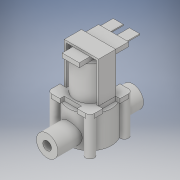
# Autodesk Inventor part: Valve
Saved by Autodesk Inventor 2018 (Build 220112000, 112)
## iProperties
Created: 2019-07-25
Part Number: Valve
Material: Generic
Document SubType Name: Modeling
Designer: micha
Density: 1 g/cm^3
Appearance: Default
Author: micha
Autodesk Inventor part; units mm, degrees
ref_plane "YZ Plane" through (0, 0, 0) normal (1, 0, 0) x (0, 1, 0)
ref_plane "XZ Plane" through (0, 0, 0) normal (0, 1, 0) x (-1, 0, 0)
ref_plane "XY Plane" through (0, 0, 0) normal (0, 0, 1) x (1, 0, 0)
sketch "Sketch1" plane through (0, 0, 0) normal (0, 0, 1) x (1, 0, 0)
  circle A0 centre (0, 0) radius 7.9375
  circle A1 centre (0, 0) radius 3.175
  dimension "d0" = 15.875
  dimension "d1" = 6.35
  constraints: 2 centre point, 2 coincident
  measures "d0" diameter of A0
  measures "d1" diameter of A1
extrude "Extrusion1" add sketch "Sketch1" along normal blind 63.5
sketch "Sketch2" plane through (0, 0, 63.5) normal (0, 0, 1) x (1, 0, 0)
  circle A0 centre (0, 0) radius 7.9375 projected
  point P0 (0, -7.9375)
  constraints: 1 vertical alignment, 1 other
ref_plane "Work Plane1" through (0, -7.9375, 63.5) normal (0, -1, 0) x (1, 0, 0)
sketch "Sketch3" plane through (0, -7.9375, 63.5) normal (0, -1, 0) x (1, 0, 0)
  line L0 (7.9375, 0) -> (-7.9375, 0) projected
  line L1 (0, 0) -> (0, -63.5) construction
  line L2 (-7.9375, -63.5) -> (7.9375, -63.5) projected
  circle A0 centre (0, -31.75) radius 15.875
  dimension "d4" = 31.75
  dimension "d5" = 31.75
  constraints: 2 end point, 2 midpoint, 1 centre point, 1 coincident, 1 vertical
  measures "d4" distance from line of L2 point (0, -31.75)
  measures "d5" diameter of A0
extrude "Extrusion2" add sketch "Sketch3" against normal blind 23.8125
sketch "Sketch4" plane through (0, 15.875, 31.75) normal (0, 1, 0) x (1, 0, 0)
  line L0 (-12.7, -12.7) -> (12.7, -12.7)
  line L1 (12.7, -12.7) -> (12.7, 12.7)
  line L2 (12.7, 12.7) -> (-12.7, 12.7)
  line L3 (-12.7, 12.7) -> (-12.7, -12.7)
  circle A0 centre (0, 0) radius 15.875 projected
  line L4 (-12.7, 6.35) -> (-12.7, -6.35)
  line L5 (-12.7, -6.35) -> (-15.875, -6.35)
  line L6 (-15.875, -6.35) -> (-15.875, -12.7)
  line L7 (-12.7, -15.875) -> (-6.35, -15.875)
  line L8 (-6.35, -15.875) -> (-6.35, -12.7)
  line L9 (-12.7, 6.35) -> (-15.875, 6.35)
  line L10 (-15.875, 6.35) -> (-15.875, 12.7)
  line L11 (-12.7, 15.875) -> (-6.35, 15.875)
  line L12 (-6.35, 15.875) -> (-6.35, 12.7)
  line L13 (6.35, 12.7) -> (6.35, 15.875)
  line L14 (6.35, 15.875) -> (12.7, 15.875)
  line L15 (15.875, 12.7) -> (15.875, 6.35)
  line L16 (15.875, 6.35) -> (12.7, 6.35)
  line L17 (6.35, -12.7) -> (6.35, -15.875)
  line L18 (6.35, -15.875) -> (12.7, -15.875)
  line L19 (15.875, -12.7) -> (15.875, -6.35)
  line L20 (15.875, -6.35) -> (12.7, -6.35)
  arc A1 (-15.875, -12.7) -> (-12.7, -15.875) centre (-12.7, -12.7) ccw
  arc A2 (-12.7, 15.875) -> (-15.875, 12.7) centre (-12.7, 12.7) ccw
  arc A3 (15.875, 12.7) -> (12.7, 15.875) centre (12.7, 12.7) ccw
  arc A4 (12.7, -15.875) -> (15.875, -12.7) centre (12.7, -12.7) ccw
  point P0 (0, 31.75)
  point P1 (-15.875, -15.875)
  point P2 (-15.875, 15.875)
  point P3 (15.875, 15.875)
  point P4 (15.875, -15.875)
  dimension "d8" = 25.4
  dimension "d9" = 25.4
  dimension "d10" = 12.7
  dimension "d11" = 12.7
  dimension "d12" = 6.35
  dimension "d13" = 12.7
  dimension "d14" = 3.175
  dimension "d15" = 9.525
  dimension "d16" = 9.525
  dimension "d17" = 9.525
  dimension "d18" = 19.05
  dimension "d19" = 3.175
  dimension "d20" = 12.7
  dimension "d21" = 9.525
  dimension "d22" = 3.175
  dimension "d23" = 9.525
  dimension "d24" = 12.7
  dimension "d25" = 9.525
  dimension "d26" = 3.175
  constraints: 42 end point, 18 point on line, 14 perpendicular, 9 tangent, 8 point on circle, 4 centre point, 3 equal radius, 3 horizontal, 2 parallel
  measures "d8" distance of L2.end L1.end
  measures "d9" distance of L1.end L0.end
  measures "d10" distance from line of L2 A0.centre
  measures "d11" distance from line of L1 A0.centre
  measures "d12" vertical distance of A0.centre L4.start
  measures "d13" distance of L4.start L4.end
  measures "d14" distance of L4.end L5.end
  measures "d15" distance of L5.end point (-15.875, -15.875)
  measures "d16" distance of point (-15.875, -15.875) L7.end
  measures "d17" distance of L9.end point (-15.875, 15.875)
  measures "d18" distance between parallel lines of L12 L1
  measures "d19" distance of L13.start L13.end
  measures "d20" distance between parallel lines of L13 L12
  measures "d21" distance of L13.end point (15.875, 15.875)
  measures "d22" distance of L17.start L17.end
  measures "d23" distance between parallel lines of L15 L17
  measures "d24" distance between parallel lines of L16 L20
  measures "d25" distance between parallel lines of L16 L14
  measures "d26" radius of A1
extrude "Extrusion3" add sketch "Sketch4" along normal blind 3.175 contours L0 A0 L3 L2 L1 | L8 A0 L0 | L0 A0 L17 | A0 L8 L7 A1 L6 L5 L3 L0 | L0 L3 A0 | A0 L1 L0 | L0 L1 A0 L20 L19 A4 L18 L17 | A0 L5 L3 | L1 L20 A0 | L9 A0 L3 | L9 L10 A2 L11 L12 A0 L2 L3 | L1 A0 L16 | L3 L2 A0 | A0 L2 L1 | L1 L2 A0 L13 L14 A3 L15 L16 | A0 L12 L2 | L2 L13 A0
sketch "Sketch5" plane through (0, 15.875, 31.75) normal (0, -1, 0) x (1, 0, 0)
  arc A0 (-15.875, -12.7) -> (-12.7, -15.875) centre (-12.7, -12.7) ccw projected
  arc A1 (12.7, -15.875) -> (15.875, -12.7) centre (12.7, -12.7) ccw projected
  arc A2 (15.875, 12.7) -> (12.7, 15.875) centre (12.7, 12.7) ccw projected
  arc A3 (-12.7, 15.875) -> (-15.875, 12.7) centre (-12.7, 12.7) ccw projected
  circle A4 centre (-12.7, 12.7) radius 3.175
  line L0 (-15.875, -12.7) -> (-15.875, -6.35) projected
  circle A5 centre (-12.7, -12.7) radius 3.175
  circle A6 centre (12.7, -12.7) radius 3.175
  circle A7 centre (12.7, 12.7) radius 3.175
  point P0 (0, -31.75)
  constraints: 4 coincident, 3 horizontal alignment, 1 centre point, 1 concentric, 6 other
extrude "Extrusion4" add sketch "Sketch5" along normal blind 25.4
sketch "Sketch6" plane through (0, 19.05, 31.75) normal (0, 1, 0) x (1, 0, 0)
  circle A0 centre (0, 0) radius 11.1125
  point P0 (0, 31.75)
  dimension "d31" = 22.225
  constraints: 1 centre point
  measures "d31" diameter of A0
extrude "Extrusion5" add sketch "Sketch6" along normal blind 25.4
sketch "Sketch7" plane through (0, 44.45, 31.75) normal (0, 1, 0) x (1, 0, 0)
  circle A0 centre (0, 0) radius 11.1125 projected
  line L0 (-6.35, 0) -> (6.35, 0)
  line L1 (6.35, 0) -> (6.35, -14.3002)
  line L2 (6.35, -14.3002) -> (-6.35, -14.3002)
  line L3 (-6.35, -14.3002) -> (-6.35, 0)
  circle A1 centre (0, 0) radius 11.1125 projected
  line L4 (11.1125, 0) -> (-11.1125, 0)
  line L5 (-11.1125, 0) -> (-11.1125, 17.4752)
  line L6 (-11.1125, 17.4752) -> (11.1125, 17.4752)
  line L7 (11.1125, 17.4752) -> (11.1125, 0)
  point P0 (0, 31.75)
  dimension "d34" = 6.35
  dimension "d35" = 12.7
  dimension "d36" = 14.3002
  dimension "d37" = 17.4752
  constraints: 16 end point, 4 parallel, 2 horizontal, 2 perpendicular, 1 horizontal alignment, 1 other
  measures "d34" distance of L0.start A0.centre
  measures "d35" distance of L1.end L2.end
  measures "d36" distance of L0.end L1.end
  measures "d37" distance of L4.end L5.end
extrude "Extrusion6" add sketch "Sketch7" along normal blind 3.175 contours L4 L0 A0 | A0 L5 L6 L7 | L1 L2 L3 A0 | A0 L3 L0 L1
sketch "Sketch8" plane through (0, 47.625, 31.75) normal (0, 1, 0) x (1, 0, 0)
  line L0 (-12.7, 6.35) -> (-12.7, -6.35) projected
  line L1 (15.875, -6.35) -> (12.7, -6.35) projected
  line L2 (-12.7, 6.35) -> (12.7, 6.35)
  line L3 (12.7, 6.35) -> (12.7, -6.35)
  line L4 (12.7, -6.35) -> (-12.7, -6.35)
  line L5 (-12.7, -6.35) -> (-12.7, 6.35)
  point P0 (0, 31.75)
  constraints: 8 end point, 2 parallel, 1 horizontal, 1 perpendicular
extrude "Extrusion7" add sketch "Sketch8" along normal blind 1.5875
sketch "Sketch9" plane through (0, 19.05, 31.75) normal (0, 1, 0) x (1, 0, 0)
  line L0 (-6.35, -6.35) -> (-12.7, -6.35) projected
  line L1 (-11.1125, 6.35) -> (-11.1125, 0) projected
  line L2 (-12.7, -6.35) -> (-11.1125, -6.35)
  line L3 (-11.1125, -6.35) -> (-11.1125, 6.35)
  line L4 (-11.1125, 6.35) -> (-12.7, 6.35)
  line L5 (-12.7, 6.35) -> (-12.7, -6.35)
  line L6 (-12.7, -6.35) -> (12.7, -6.35) projected
  line L7 (12.7466, 6.35) -> (11.1591, 6.35)
  line L8 (11.1591, 6.35) -> (11.1591, -6.35)
  line L9 (11.1591, -6.35) -> (12.7466, -6.35)
  line L10 (12.7466, -6.35) -> (12.7466, 6.35)
  point P0 (0, 31.75)
  dimension "d42" = 1.5875
  dimension "d43" = 1.5875
  constraints: 16 end point, 4 parallel, 2 horizontal, 2 perpendicular, 2 point on line
  measures "d42" distance of L4.end L1.start
  measures "d43" distance of L9.end L8.end
extrude "Extrusion8" add sketch "Sketch9" along normal blind 30.1625
sketch "Sketch10" plane through (11.1125, 44.45, 14.2748) normal (0, 0, -1) x (-1, 0, 0)
  line L0 (20.955, 2.921) -> (13.335, 2.921)
  line L1 (13.335, 2.921) -> (13.335, 2.159)
  line L2 (13.335, 2.159) -> (20.955, 2.159)
  line L3 (20.955, 2.159) -> (20.955, 2.921)
  line L4 (8.89, 2.921) -> (1.27, 2.921)
  line L5 (1.27, 2.921) -> (1.27, 2.159)
  line L6 (1.27, 2.159) -> (8.89, 2.159)
  line L7 (8.89, 2.159) -> (8.89, 2.921)
  line L8 (22.225, 0) -> (22.225, 3.175) projected
  line L9 (0, 0) -> (0, 3.175) projected
  line L10 (0, 3.175) -> (22.225, 3.175) projected
  point P0 (11.1125, -44.45)
  dimension "d46" = 1.27
  dimension "d47" = 7.62
  dimension "d48" = 1.27
  dimension "d49" = 7.62
  dimension "d50" = 0.254
  dimension "d51" = 0.762
  constraints: 16 end point, 4 parallel, 2 horizontal, 2 perpendicular, 2 point on line
  measures "d46" distance between parallel lines of L8 L3
  measures "d47" distance between parallel lines of L3 L1
  measures "d48" distance between parallel lines of L9 L5
  measures "d49" distance of L4.start L4.end
  measures "d50" distance between parallel lines of L10 L4
  measures "d51" distance between parallel lines of L0 L2
extrude "Extrusion9" add sketch "Sketch10" along normal blind 9.525
body "Solid1"
